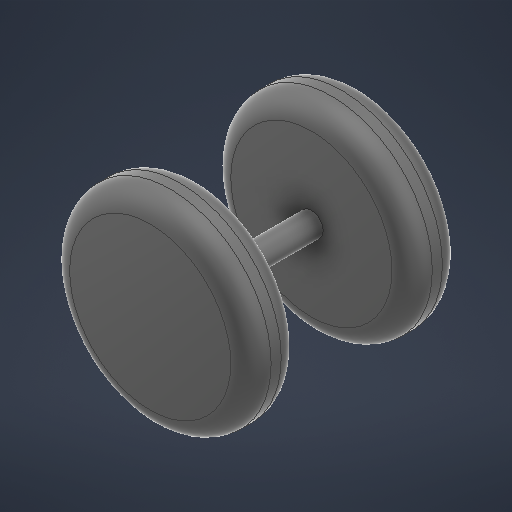
# Autodesk Inventor part: WHEEL
Saved by Autodesk Inventor 2027.1 (Build 311270010, 270A)
## iProperties
Created: 2026-08-29
Part Number: WHEEL
Material: Generic
Document SubType Name: Modeling
Designer: RIDDHIMAN
Density: 1 g/cm^3
Appearance: Default
Author: RIDDHIMAN
Autodesk Inventor part; units mm, degrees
ref_plane "YZ Plane" through (0, 0, 0) normal (1, 0, 0) x (0, 1, 0)
ref_plane "XZ Plane" through (0, 0, 0) normal (0, 1, 0) x (-1, 0, 0)
ref_plane "XY Plane" through (0, 0, 0) normal (0, 0, 1) x (1, 0, 0)
sketch "Sketch1" plane through (0, 0, 0) normal (0, 1, 0) x (-1, 0, 0)
  line L0 (-50, -27.5) -> (-50, -52.5)
  line L1 (-50, -52.5) -> (0, -52.5)
  line L2 (0, 52.5) -> (-50, 52.5)
  line L3 (-50, 52.5) -> (-50, 27.5)
  line L4 (-50, 27.5) -> (-5.8866, 27.5)
  line L5 (-5.8866, -27.5) -> (-50, -27.5)
  line L6 (-5.8866, 27.5) -> (-5.8866, -27.5)
  line L7 (0, -52.5) -> (0, 52.5)
  point P0 (0, 0)
  constraints: 16 end point, 2 horizontal, 2 parallel, 2 perpendicular
revolve "Revolution1" add sketch "Sketch1" angle 360 about axis through (0, 0, -52.5) along (0, 0, 1)
fillet "Fillet1" radius 10 4 edges at (-50, 0, 27.5) (-50, 0, -27.5) (-50, 0, -52.5) (-50, 0, 52.5)
body "Solid1"
